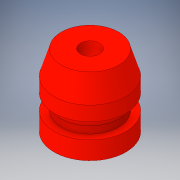
# Autodesk Inventor part: modular-post
Saved by Autodesk Inventor 2017 (Build 210142000, 142)
## iProperties
Created: 2017-02-19
Part Number: modular-post
Material: Generic
Document SubType Name: Modeling
Designer: John
Density: 1 g/cm^3
Appearance: Default
Author: John
Autodesk Inventor part; units mm, degrees
ref_plane "YZ Plane" through (0, 0, 0) normal (1, 0, 0) x (0, 1, 0)
ref_plane "XZ Plane" through (0, 0, 0) normal (0, 1, 0) x (-1, 0, 0)
ref_plane "XY Plane" through (0, 0, 0) normal (0, 0, 1) x (1, 0, 0)
sketch "Sketch3" plane through (0, 0, 0) normal (0, 0, 1) x (1, 0, 0)
  line L0 (0, 0) -> (10, 0)
  line L1 (0, 0) -> (0, 20)
  line L2 (0, 20) -> (8, 20)
  line L3 (10, 0) -> (10, 5)
  line L4 (10, 5) -> (8, 5)
  line L5 (8, 5) -> (8, 7)
  line L6 (8, 7) -> (10, 9.3965)
  line L7 (10, 9.3965) -> (10, 13.3965)
  line L8 (10, 13.3965) -> (8, 20)
  dimension "d17" = 10
  dimension "d18" = 20
  dimension "d19" = 8
  dimension "d40" = 5
  dimension "d43" = 2
  dimension "d44" = 4
  dimension "d45" = 2
  constraints: 18 end point, 3 vertical, 2 horizontal, 2 parallel, 1 collinear
  measures "d17" distance of L0.start L0.end
  measures "d18" distance of L0.start L1.end
  measures "d19" distance of L1.end L2.end
  measures "d40" distance of L0.end L3.end
  measures "d43" distance of L4.end L5.end
  measures "d44" distance of L6.end L7.end
  measures "d45" distance of L3.end L4.end
revolve "Revolution1" add sketch "Sketch3" angle 360 about axis through (0, 0, 0) along (0, 1, 0)
sketch "Sketch4" plane through (0, 0, 0) normal (0, 1, 0) x (-1, 0, 0)
  circle A0 centre (0, 0) radius 1.5
  dimension "d27" = 3
  constraints: 1 centre point, 1 coincident
  measures "d27" diameter of A0
extrude "Extrusion3" cut sketch "Sketch4" along normal through all
sketch "Sketch5" plane through (0, 20, 0) normal (0, 1, 0) x (1, 0, 0)
  circle A0 centre (0, 0) radius 2.65
  dimension "d30" = 5.3
  constraints: 1 centre point, 1 coincident
  measures "d30" diameter of A0
extrude "Extrusion4" cut sketch "Sketch5" against normal blind 5
sketch "Sketch6" plane through (0, 0, 0) normal (0, -1, 0) x (1, 0, 0)
  circle A0 centre (-6, 0) radius 1.5
  circle A1 centre (6, 0) radius 1.5
  circle A2 centre (0, 0) radius 1.5 projected
  line L0 (-6, 0) -> (0, 0) construction
  line L1 (0, 0) -> (6, 0) construction
  dimension "d33" = 3
  dimension "d35" = 3
  dimension "d47" = 6
  constraints: 4 end point, 2 centre point, 2 collinear, 1 horizontal
  measures "d33" diameter of A0
  measures "d35" diameter of A1
  measures "d47" distance of L0.end L1.end
extrude "Extrusion5" [suppressed]
equation "\"d35\" = d33"
equation "\"d47\" = 2 * d33"
body "Solid2"
